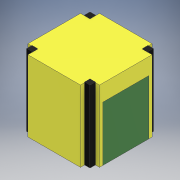
# Autodesk Inventor part: CubeSatStandard
Saved by Autodesk Inventor 2018 (Build 220112000, 112)
## iProperties
Created: 2018-07-04
Part Number: CubeSatStandard
Material: Aluminum 6061
Document SubType Name: Modeling
Designer: Bradley
Density: 2.7 g/cm^3
Appearance: Anodized - Dark Gray
Author: Bradley
Autodesk Inventor part; units mm, degrees
ref_plane "YZ Plane" through (0, 0, 0) normal (1, 0, 0) x (0, 1, 0)
ref_plane "XZ Plane" through (0, 0, 0) normal (0, 1, 0) x (-1, 0, 0)
ref_plane "XY Plane" through (0, 0, 0) normal (0, 0, 1) x (1, 0, 0)
sketch "Sketch1" plane through (0, 0, 0) normal (0, 0, 1) x (1, 0, 0)
  line L0 (50, -50) -> (-50, -50)
  line L1 (-50, -50) -> (-50, 50)
  line L2 (-50, 50) -> (50, 50)
  line L3 (50, 50) -> (50, -50)
  line L4 (50, -50) -> (-50, 50) construction
  line L5 (-50, -50) -> (50, 50) construction
  line L6 (-50, -41.5) -> (-56.5, -41.5)
  line L7 (-56.5, -41.5) -> (-56.5, 41.5)
  line L8 (-56.5, 41.5) -> (-50, 41.5)
  line L9 (-50, 41.5) -> (-50, -41.5)
  line L10 (-41.5, 50) -> (41.5, 50)
  line L11 (41.5, 50) -> (41.5, 56.5)
  line L12 (41.5, 56.5) -> (-41.5, 56.5)
  line L13 (-41.5, 56.5) -> (-41.5, 50)
  line L14 (50, 41.5) -> (56.5, 41.5)
  line L15 (56.5, 41.5) -> (56.5, -41.5)
  line L16 (56.5, -41.5) -> (50, -41.5)
  line L17 (50, -41.5) -> (50, 41.5)
  line L18 (41.5, -50) -> (-41.5, -50)
  line L19 (-41.5, -50) -> (-41.5, -56.5)
  line L20 (-41.5, -56.5) -> (41.5, -56.5)
  line L21 (41.5, -56.5) -> (41.5, -50)
  point P0 (0, 0)
  point P1 (-50, 0)
  point P2 (0, 50)
  point P3 (50, 0)
  point P4 (0, -50)
  dimension "d0" = 100
  dimension "d1" = 6.5
  dimension "d2" = 8.5
  constraints: 44 end point, 10 midpoint, 10 parallel, 10 perpendicular, 8 point on line, 5 horizontal
  measures "d0" distance of L1.end L2.end
  measures "d1" distance of L6.start L6.end
  measures "d2" distance between parallel lines of L6 L0
extrude "Extrusion1" add sketch "Sketch1" along normal blind 57 and the other way blind 56.5
sketch "Sketch2" plane through (0, 0, 57) normal (0, 0, 1) x (1, 0, 0)
  line L0 (-41.5, -50) -> (-41.5, -56.5) projected
  line L1 (-41.5, -56.5) -> (41.5, -56.5) projected
  line L2 (41.5, -56.5) -> (41.5, -50) projected
  line L3 (41.5, -50) -> (50, -50) projected
  line L4 (50, -50) -> (50, -41.5) projected
  line L5 (50, -41.5) -> (56.5, -41.5) projected
  line L6 (56.5, -41.5) -> (56.5, 41.5) projected
  line L7 (56.5, 41.5) -> (50, 41.5) projected
  line L8 (50, 41.5) -> (50, 50) projected
  line L9 (50, 50) -> (41.5, 50) projected
  line L10 (41.5, 50) -> (41.5, 56.5) projected
  line L11 (41.5, 56.5) -> (-41.5, 56.5) projected
  line L12 (-41.5, 56.5) -> (-41.5, 50) projected
  line L13 (-41.5, 50) -> (-50, 50) projected
  line L14 (-50, 50) -> (-50, 41.5) projected
  line L15 (-50, 41.5) -> (-56.5, 41.5) projected
  line L16 (-56.5, 41.5) -> (-56.5, -41.5) projected
  line L17 (-56.5, -41.5) -> (-50, -41.5) projected
  line L18 (-50, -41.5) -> (-50, -50) projected
  line L19 (-50, -50) -> (-41.5, -50) projected
  line L20 (-50, -41.5) -> (-50, -50) projected
  line L21 (-50, -41.5) -> (-41.5, -41.5)
  line L22 (-41.5, -41.5) -> (-41.5, -50)
  line L23 (-50, 50) -> (-50, 41.5) projected
  line L24 (-50, 41.5) -> (-41.5, 41.5)
  line L25 (-41.5, 41.5) -> (-41.5, 50)
  line L26 (41.5, 56.5) -> (41.5, 50) projected
  line L27 (41.5, 50) -> (41.5, 41.5)
  line L28 (41.5, 41.5) -> (50, 41.5)
  line L29 (41.5, -50) -> (41.5, -41.5)
  line L30 (50, -41.5) -> (56.5, -41.5) projected
  line L31 (50, -41.5) -> (41.5, -41.5)
  point P0 (0, 0)
  constraints: 16 end point, 4 perpendicular, 4 point on line, 2 collinear, 1 horizontal
extrude "Extrusion2" cut sketch "Sketch2" against normal blind 1 contours L22 L21 L17 L16 L15 L24 L25 L12 L11 L10 L27 L28 L7 L6 L5 L31 L29 L2 L1 L0
sketch "Sketch3" plane through (56.5, -41.5, -56.5) normal (1, 0, 0) x (0, 0, -1)
  line L0 (-112.5, 83) -> (-112.5, 0) projected
  line L1 (0, 0) -> (-112.5, 0) projected
  line L2 (0, 83) -> (0, 0) projected
  line L3 (0, 83) -> (-112.5, 83) projected
  line L4 (-86.5, 5.25) -> (0, 5.25)
  line L5 (0, 5.25) -> (0, 77.75)
  line L6 (0, 77.75) -> (-86.5, 77.75)
  line L7 (-86.5, 77.75) -> (-86.5, 5.25)
  line L8 (0, 83) -> (0, 0) projected
  point P0 (-56.5, 41.5)
  point P1 (0, 41.5)
  dimension "d9" = 72.5
  dimension "d10" = 86.5
  constraints: 8 end point, 2 midpoint, 2 parallel, 1 collinear, 1 horizontal, 1 perpendicular
  measures "d9" distance of L6.end L4.start
  measures "d10" distance of L5.end L6.end
split_face "Split1"
sketch "Sketch4" plane through (0, 0, -56.5) normal (0, 0, -1) x (-1, 0, 0)
  line L0 (41.5, -56.5) -> (41.5, -50) projected
  line L1 (-41.5, -56.5) -> (41.5, -56.5) projected
  line L2 (-41.5, -50) -> (-41.5, -56.5) projected
  line L3 (-41.5, -41.5) -> (-41.5, -50) projected
  line L4 (-50, -41.5) -> (-41.5, -41.5) projected
  line L5 (-56.5, -41.5) -> (-50, -41.5) projected
  line L6 (-56.5, 41.5) -> (-56.5, -41.5) projected
  line L7 (-50, 41.5) -> (-56.5, 41.5) projected
  line L8 (-41.5, 41.5) -> (-50, 41.5) projected
  line L9 (-41.5, 50) -> (-41.5, 41.5) projected
  line L10 (-41.5, 56.5) -> (-41.5, 50) projected
  line L11 (41.5, 56.5) -> (-41.5, 56.5) projected
  line L12 (41.5, 50) -> (41.5, 56.5) projected
  line L13 (41.5, 41.5) -> (41.5, 50) projected
  line L14 (50, 41.5) -> (41.5, 41.5) projected
  line L15 (56.5, 41.5) -> (50, 41.5) projected
  line L16 (56.5, -41.5) -> (56.5, 41.5) projected
  line L17 (50, -41.5) -> (56.5, -41.5) projected
  line L18 (41.5, -41.5) -> (50, -41.5) projected
  line L19 (41.5, -50) -> (41.5, -41.5) projected
  point P0 (0, 0)
split_face "Split2"
body "Solid1"
